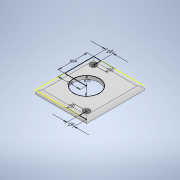
# Autodesk Inventor part: sample holder lid for neutron r1
Saved by Autodesk Inventor 2020 (Build 240168000, 168)
## iProperties
Created: 2022-04-13
Part Number: sample holder lid for neutron r1
Material: Generic
Document SubType Name: Modeling
Designer: Beaucage
Density: 1 g/cm^3
Appearance: Default
Author: Beaucage
Autodesk Inventor part; units mm, degrees
ref_plane "YZ Plane" through (0, 0, 0) normal (1, 0, 0) x (0, 1, 0)
ref_plane "XZ Plane" through (0, 0, 0) normal (0, 1, 0) x (-1, 0, 0)
ref_plane "XY Plane" through (0, 0, 0) normal (0, 0, 1) x (1, 0, 0)
sketch "Sketch1" plane through (0, 0, 0) normal (0, 1, 0) x (-1, 0, 0)
  line L0 (0, 0) -> (44.45, 0)
  line L1 (44.45, 0) -> (44.45, -50.4952)
  line L2 (44.45, -50.4952) -> (0, -50.4952)
  line L3 (0, -50.4952) -> (0, 0)
  dimension "d0" = 44.45
  dimension "d1" = 50.4952
  constraints: 8 end point, 2 parallel, 1 horizontal, 1 perpendicular
  measures "d0" distance of L1.end L2.end
  measures "d1" distance of L0.end L1.end
extrude "Extrusion1" add sketch "Sketch1" along normal blind 3.175
sketch "Sketch2" plane through (0, 3.175, 0) normal (0, 1, 0) x (1, 0, 0)
  line L0 (-44.45, 50.4952) -> (-44.45, 0) projected
  line L1 (-44.45, 50.4952) -> (-38.1, 50.4952)
  line L2 (0, 50.4952) -> (-44.45, 50.4952) projected
  line L3 (-38.1, 50.4952) -> (-38.1, 44.1452)
  line L4 (-44.45, 0) -> (0, 0) projected
  line L5 (0, 0) -> (-6.35, 0)
  line L6 (-6.35, 0) -> (-6.35, 6.35)
  line L7 (-44.45, 50.4952) -> (-44.45, 25.2476)
  line L8 (-44.45, 25.2476) -> (-25.4, 25.2476)
  circle A0 centre (-25.4, 25.2476) radius 11.1125
  dimension "d4" = 6.35
  dimension "d5" = 6.35
  dimension "d6" = 6.35
  dimension "d7" = 6.35
  dimension "d15" = 25.2476
  dimension "d16" = 19.05
  dimension "d17" = 22.225
  constraints: 12 end point, 3 perpendicular, 2 point on line, 1 centre point, 1 coincident, 1 midpoint
  measures "d4" distance of L0.start L1.end
  measures "d5" distance of L1.end L3.end
  measures "d6" distance of L4.end L5.end
  measures "d7" distance of L5.end L6.end
  measures "d15" distance of L0.start L7.end
  measures "d16" distance of L7.end L8.end
  measures "d17" diameter of A0
hole "Hole1" at (-6.35, 3.175, -6.35) at (-38.1, 3.175, -44.1452) direction (0, -1, 0) diameter 3.2766 depth 12.7 tip angle 118 counterbore diameter 5.5626 counterbore depth 1.5875 clearance for "Socket Head Cap Screw" size "#4" standard "Ansi Unified Screw Threads"
extrude "Extrusion2" cut sketch "Sketch2" against normal blind 3.175
fillet "Fillet1" radius 3.175 4 edges at (-44.45, 3.175, -25.2476) (-22.225, 3.175, -50.4952) (0, 3.175, -25.2476) (-22.225, 3.175, 0)
body "Solid1"
